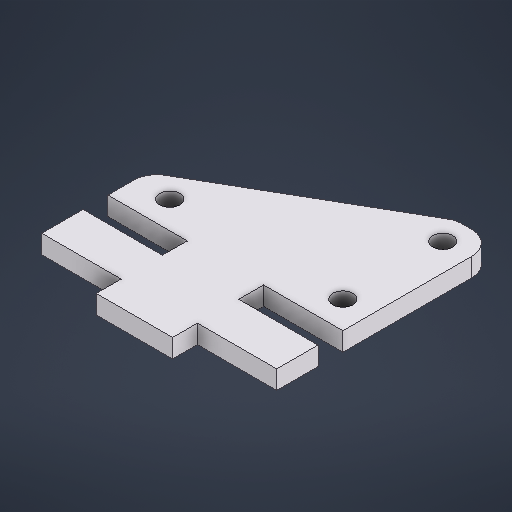
# Autodesk Inventor part: INTAKE_BACK_MOUNT_PLATE
Saved by Autodesk Inventor 2026.2 (Build 302298010, 298A)
## iProperties
Created: 2026-04-02
Part Number: INTAKE_BACK_MOUNT_PLATE
Material: Aluminum, 6061-T6
Document SubType Name: Sheet Metal
Designer: 4aida
Density: 2.71 g/cm^3
Sheet Metal Rule: Default_mm
Appearance: Metal-AL-6061 (Flat)
Author: 4aida
Autodesk Inventor part; units mm, degrees
ref_plane "YZ Plane" through (0, 0, 0) normal (1, 0, 0) x (0, 1, 0)
ref_plane "XZ Plane" through (0, 0, 0) normal (0, 1, 0) x (-1, 0, 0)
ref_plane "XY Plane" through (0, 0, 0) normal (0, 0, 1) x (1, 0, 0)
sketch "Sketch1" plane through (0, 0, 0) normal (0, 1, 0) x (-1, 0, 0)
  line L0 (-30, -11.6205) -> (30, -11.6205)
  line L1 (30, -11.6205) -> (30, 11.6205)
  line L2 (30, 11.6205) -> (-30, 11.6205)
  line L3 (-30, 11.6205) -> (-30, -11.6205)
  line L4 (-30, -11.6205) -> (30, 11.6205) construction
  line L5 (30, -11.6205) -> (-30, 11.6205) construction
  line L6 (-9.746, 11.6205) -> (-9.746, 5.2705)
  line L7 (-9.746, 5.2705) -> (-30, 5.2705)
  line L8 (30, 5.2705) -> (9.746, 5.2705)
  line L9 (9.746, 5.2705) -> (9.746, 11.6205)
  line L10 (30, 0) -> (0, 0) construction
  line L11 (-9.746, -11.6205) -> (-9.746, -5.2705)
  line L12 (-9.746, -5.2705) -> (-30, -5.2705)
  line L13 (30, -5.2705) -> (9.746, -5.2705)
  line L14 (9.746, -5.2705) -> (9.746, -11.6205)
  line L15 (30, -11.6205) -> (30, -21.6205)
  line L16 (30, -21.6205) -> (-20, -50.488)
  line L17 (-20, -50.488) -> (-30, -50.488)
  line L18 (-30, -50.488) -> (-30, -11.6205)
  dimension "d0" = 20.254
  dimension "d1" = 20.254
  dimension "d2" = 6.35
  dimension "d3" = 60
  dimension "d4" = 23.241
  dimension "d5" = 10
  dimension "d6" = 10
  dimension "d7" = 60
  measures "d0" distance between parallel lines of L1 L9
  measures "d1" distance between parallel lines of L3 L6
  measures "d2" distance of L6.start L6.end
  measures "d3" distance of L1.end L2.end
  measures "d4" distance of L0.end L1.end
  measures "d5" distance of L16.end L17.end
  measures "d6" distance of L0.end L15.end
  measures "d7" angle of L18 L16
extrude "Plate1" add sketch "Sketch1" along normal blind 4.7625 contours L0 L15 L16 L17 L18 | L11 L12 L3 L7 L6 L2 L9 L8 L1 L13 L14 L0
fillet "Corner Round1" radius 6 3 edges at (-30, 2.3813, -21.6205) (20, 2.3813, -50.488) (30, 2.3813, -50.488)
sketch "Sketch2" plane through (0, 4.7625, 0) normal (0, 1, 0) x (1, 0, 0)
  line L0 (-21.1962, 18.6205) -> (23, 18.6205)
  line L1 (23, 18.6205) -> (23, 44.1372)
  line L2 (23, 44.1372) -> (-21.1962, 18.6205)
  line L3 (-27, 23.3526) -> (18.6077, 49.6842) projected
  line L4 (-9.746, 11.6205) -> (-30, 11.6205) projected
  line L5 (30, 44.488) -> (30, 11.6205) projected
  point P0 (0, 0)
  dimension "d10" = 7
  dimension "d11" = 7
  dimension "d12" = 7
  constraints: 6 end point, 1 horizontal, 1 parallel, 1 perpendicular
  measures "d10" distance between parallel lines of L4 L0
  measures "d11" distance between parallel lines of L5 L1
  measures "d12" distance between parallel lines of L3 L2
hole "Hole1" at (-21.1962, 4.7625, -18.6205) at (23, 4.7625, -18.6205) at (23, 4.7625, -44.1372) direction (0, -1, 0) diameter 5.105 end through all clearance for "Socket Head Cap Screw" size "#10" standard "Ansi Unified Screw Threads"
equation "\"d1\" = d0"
equation "\"d6\" = d5"
equation "\"d11\" = d10"
equation "\"d12\" = d10"
equation "\"d18\" = Thickness"
equation "\"d8\" = Thickness"
equation "\"BendRadius\" = Thickness"
equation "\"BendReliefWidth\" = Thickness"
equation "\"BendReliefDepth\" = 0.5 * Thickness"
equation "\"CornerReliefSize\" = 4 * Thickness"
equation "\"MinimumRemnant\" = 2 * Thickness"
equation "\"TransitionRadius\" = BendRadius"
equation "\"JacobiRadiusSize\" = BendRadius"
equation "\"GapSize\" = Thickness"
equation "\"Thickness\" = 4.7625"
body "Solid1"
